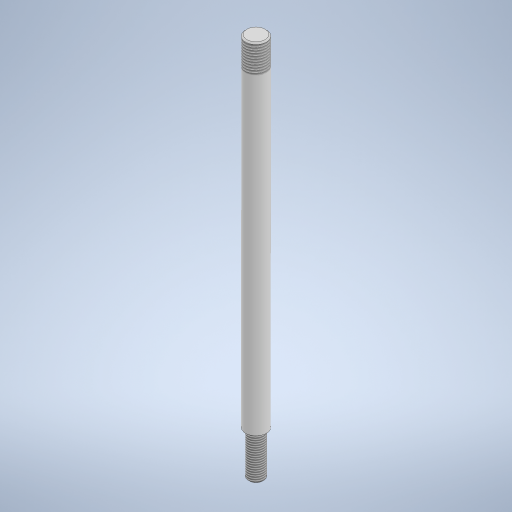
# Autodesk Inventor part: BARRA SOPORTE
Saved by Autodesk Inventor 2024.1 (Build 281209000, 209)
## iProperties
Created: 2025-06-24
Part Number: BARRA SOPORTE
Material: Generic
Document SubType Name: Modeling
Designer: User
Density: 1 g/cm^3
Appearance: Default
Author: User
Autodesk Inventor part; units mm, degrees
ref_plane "YZ Plane" through (0, 0, 0) normal (1, 0, 0) x (0, 1, 0)
ref_plane "XZ Plane" through (0, 0, 0) normal (0, 1, 0) x (-1, 0, 0)
ref_plane "XY Plane" through (0, 0, 0) normal (0, 0, 1) x (1, 0, 0)
sketch "Sketch1" plane through (0, 0, 0) normal (0, 1, 0) x (-1, 0, 0)
  circle A0 centre (0, 0) radius 15
  dimension "d0" = 30
  constraints: 1 centre point, 1 coincident
  measures "d0" diameter of A0
extrude "Extrusion1" add sketch "Sketch1" along normal blind 459
sketch "Sketch2" plane through (0, 0, 0) normal (0, -1, 0) x (1, 0, 0)
  circle A0 centre (0, 0) radius 11
  dimension "d3" = 22
  constraints: 1 centre point, 1 coincident
  measures "d3" diameter of A0
extrude "Extrusion2" add sketch "Sketch2" along normal blind 62
fillet "Fillet1" radius 2 1 edges at (-11, 0, 0)
sketch "Sketch3" plane through (0, 459, 0) normal (0, 1, 0) x (1, 0, 0)
  circle A0 centre (0, 0) radius 15
  dimension "d7" = 30
  constraints: 1 centre point, 1 coincident
  measures "d7" diameter of A0
extrude "Extrusion3" add sketch "Sketch3" along normal blind 12.7
thread "Thread2" size "M22x3" class "6g" standard "ANSI Metric M Profile" length 60
sketch "Sketch4" plane through (0, 471.7, 0) normal (0, 1, 0) x (1, 0, 0)
  circle A0 centre (0, 0) radius 15 projected
extrude "Extrusion4" add sketch "Sketch4" along normal blind 12
thread "Thread3" size "M30x3.5" class "6g" standard "ANSI Metric M Profile" length 40
chamfer "Chamfer1" distance 2 angle 45 1 edges at (-15, 483.7, 0)
chamfer "Chamfer2" distance 2 angle 45 1 edges at (-11, -62, 0)
body "Solid1"
